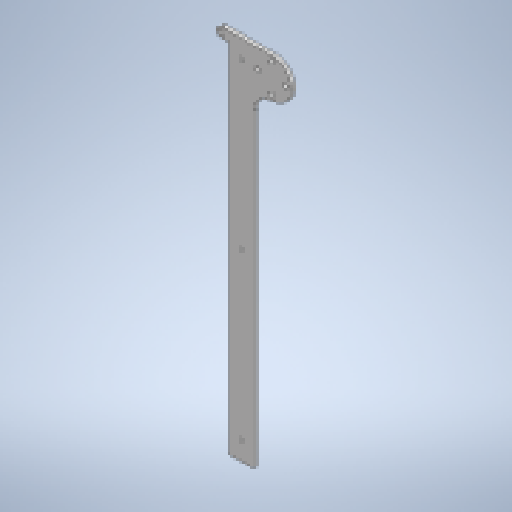
# Autodesk Inventor part: ServoMountPlate
Saved by Autodesk Inventor 2023 (Build 270158000, 158)
## iProperties
Created: 2022-09-10
Part Number: ServoMountPlate
Material: Generic
Document SubType Name: Modeling
Designer: deli
Density: 1 g/cm^3
Appearance: Default
Mass: 21.7862 g
Surface Area: 161.445 cm^2
Volume: 21.7862 cm^3
Author: deli
Autodesk Inventor part; units mm, degrees
ref_plane "YZ Plane" through (0, 0, 0) normal (1, 0, 0) x (0, 1, 0)
ref_plane "XZ Plane" through (0, 0, 0) normal (0, 1, 0) x (-1, 0, 0)
ref_plane "XY Plane" through (0, 0, 0) normal (0, 0, 1) x (1, 0, 0)
sketch "Sketch1" plane through (0, 0, 0) normal (0, 0, 1) x (1, 0, 0)
  circle A0 centre (142.2291, 58.2602) radius 1.6 projected
  circle A1 centre (142.2291, -76.7398) radius 1.6 projected
  circle A2 centre (142.2291, -211.7398) radius 1.6 projected
  line L0 (132.2291, -226.7398) -> (132.2291, 73.2602) projected
  line L1 (132.2291, -226.7398) -> (152.2291, -226.7398) projected
  line L2 (152.2291, 26.1102) -> (152.2291, -226.7398)
  circle A3 centre (167.3791, 68.574) radius 2
  circle A4 centre (178.6928, 57.2602) radius 2
  circle A5 centre (156.0654, 57.2602) radius 2
  circle A6 centre (167.3791, 45.9465) radius 2
  line L3 (167.3791, 68.574) -> (156.0654, 57.2602) construction
  line L4 (156.0654, 57.2602) -> (167.3791, 45.9465) construction
  line L5 (167.3791, 45.9465) -> (178.6928, 57.2602) construction
  line L6 (178.6928, 57.2602) -> (167.3791, 68.574) construction
  line L7 (167.3791, 45.9465) -> (167.3791, 68.574) construction
  arc A7 (167.3791, 41.2602) -> (167.3791, 73.2602) centre (167.3791, 57.2602) ccw
  line L8 (132.2291, 73.2602) -> (167.3791, 73.2602)
  line L9 (118.8791, 73.2602) -> (118.8791, -226.7398)
  arc A8 (167.3791, 41.2602) -> (152.2291, 26.1102) centre (167.3791, 26.1102) ccw
  arc A9 (126.2291, 73.2602) -> (126.2291, 65.2602) centre (126.2291, 69.2602) ccw
  circle A10 centre (126.2291, 69.2602) radius 2
  line L10 (126.2291, 73.2602) -> (132.2291, 73.2602)
  arc A11 (132.2291, 64.2602) -> (131.2291, 65.2602) centre (131.2291, 64.2602) ccw
  line L11 (126.2291, 65.2602) -> (131.2291, 65.2602)
  point P0 (0, 0)
  dimension "d2" = 3.2
  dimension "d4" = 4
  dimension "d5" = 4
  dimension "d6" = 4
  dimension "d7" = 4
  dimension "d9" = 16
  dimension "d10" = 16
  dimension "d15" = 32
  dimension "d16" = 48.5
  dimension "d18" = 15.15
  dimension "d19" = 30.3
  dimension "d22" = 8
  dimension "d23" = 4
  dimension "d24" = 6
  dimension "d25" = 2
  constraints: 20 end point, 9 centre point, 8 point on circle, 7 tangent, 5 perpendicular, 2 vertical, 1 coincident, 1 collinear, 1 horizontal, 1 midpoint, 1 point on line, 2 other
  measures "d2" diameter of A0
  measures "d4" diameter of A3
  measures "d5" diameter of A6
  measures "d6" diameter of A4
  measures "d7" diameter of A5
  measures "d9" distance of L3.start L3.end
  measures "d10" distance of L5.end L3.start
  measures "d15" diameter of A7
  measures "d16" distance from line of A7.centre L9
  measures "d18" distance from line of L2 A7.centre
  measures "d19" diameter of A8
  measures "d22" diameter of A9
  measures "d23" diameter of A10
  measures "d24" distance from line of L0 A10.centre
  measures "d25" diameter of A11
extrude "Extrusion2" add sketch "Sketch1" along normal blind 3.175
equation "\"d5\" = d4"
equation "\"d6\" = d4"
equation "\"d7\" = d4"
equation "\"d10\" = d9"
equation "\"d19\" = 2 * d18"
body "Solid2"
